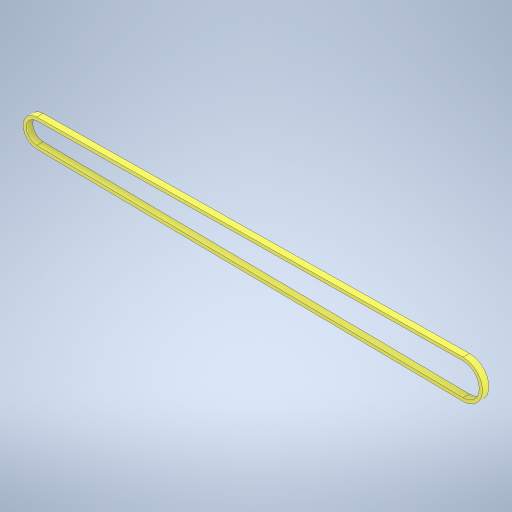
# Autodesk Inventor part: cadena
Saved by Autodesk Inventor 2023 (Build 270158030, 158C)
## iProperties
Created: 2022-05-25
Part Number: cadena
Material: Genérico
Document SubType Name: Modeling
Designer: isaac
Density: 1 g/cm^3
Appearance: Valor por defecto
Author: isaac
Autodesk Inventor part; units mm, degrees
ref_plane "YZ Plane" through (0, 0, 0) normal (1, 0, 0) x (0, 1, 0)
ref_plane "XZ Plane" through (0, 0, 0) normal (0, 1, 0) x (-1, 0, 0)
ref_plane "XY Plane" through (0, 0, 0) normal (0, 0, 1) x (1, 0, 0)
sketch "Boceto1" plane through (0, 0, 0) normal (0, 0, 1) x (1, 0, 0)
  arc A0 (-1000.625, 49.9961) -> (-1000.625, -49.9961) centre (-1000, 0) ccw
  arc A1 (999.0625, -74.9941) -> (999.0625, 74.9941) centre (1000, 0) ccw
  line L0 (999.0625, 74.9941) -> (-1000.625, 49.9961)
  line L1 (-1000.625, -49.9961) -> (999.0625, -74.9941)
  line L2 (-1000.8125, 64.9949) -> (998.875, 89.993)
  arc A2 (998.875, -89.993) -> (998.875, 89.993) centre (1000, 0) ccw
  line L3 (998.875, -89.993) -> (-1000.8125, -64.9949)
  arc A3 (-1000.8125, 64.9949) -> (-1000.8125, -64.9949) centre (-1000, 0) ccw
  point P0 (0, 0)
  dimension "d0" = 2000
  dimension "d1" = 1000
  dimension "d2" = 100
  dimension "d3" = 150
  dimension "d4" = 15
  constraints: 8 end point, 8 point on circle, 4 centre point, 4 tangent, 2 horizontal alignment, 3 other
  measures "d0" distance of A1.centre A0.centre
  measures "d1" distance of point (0, 0) A0.centre
  measures "d2" diameter of A0
  measures "d3" diameter of A1
  measures "d4" distance between parallel lines of L0 L2
extrude "Extrusión1" add sketch "Boceto1" along normal blind 30
equation "\"d1\" = 0.5 * d0"
